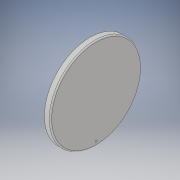
# Autodesk Inventor part: wheel hubcap
Saved by Autodesk Inventor 2019 (Build 230136000, 136)
## iProperties
Created: 2017-10-16
Part Number: wheel hubcap
Material: Generic
Document SubType Name: Modeling
Designer: M Koeppen
Density: 1 g/cm^3
Appearance: Default
Author: M Koeppen
Autodesk Inventor part; units mm, degrees
ref_plane "YZ Plane" through (0, 0, 0) normal (1, 0, 0) x (0, 1, 0)
ref_plane "XZ Plane" through (0, 0, 0) normal (0, 1, 0) x (-1, 0, 0)
ref_plane "XY Plane" through (0, 0, 0) normal (0, 0, 1) x (1, 0, 0)
sketch "Sketch5" plane through (0, 0, 0) normal (0, 0, 1) x (1, 0, 0)
  line L0 (0, 0) -> (0, 3.175)
  line L1 (0, 3.175) -> (5.715, 3.175)
  line L2 (6.35, 4.191) -> (6.35, 47.625)
  line L3 (6.35, 47.625) -> (12.7, 47.625)
  line L4 (12.7, 47.625) -> (12.7, 0)
  line L5 (12.7, 0) -> (0, 0)
  line L6 (5.715, 3.175) -> (5.715, 4.191)
  line L7 (5.715, 4.191) -> (6.35, 4.191)
  point P0 (9.525, 3.175)
  dimension "d9" = 3.175
  dimension "d10" = 47.625
  dimension "d14" = 6.35
  dimension "d18" = 0.635
  dimension "d19" = 4.191
  dimension "d21" = 5.715
  constraints: 16 end point, 5 perpendicular, 2 vertical, 1 point on line
  measures "d9" distance between parallel lines of L5 L1
  measures "d10" distance between parallel lines of L5 L3
  measures "d14" distance between parallel lines of L4 L2
  measures "d18" distance between parallel lines of L6 L2
  measures "d19" distance between parallel lines of L7 L5
  measures "d21" distance between parallel lines of L6 L0
revolve "Revolution1" add sketch "Sketch5" angle 360 about axis through (12.7, 0, 0) along (-1, 0, 0)
fillet "Fillet1" radius 1.27 1 edges at (12.7, -47.625, 0)
chamfer "Chamfer1" distance 0.635 angle 45 1 edges at (0, -3.175, 0)
sketch "Sketch6" plane through (12.7, 0, 0) normal (1, 0, 0) x (0, 0, -1)
  circle A0 centre (0, 0) radius 46.355 projected
  line L0 (-34.925, -19.05) -> (34.925, -19.05)
  line L1 (0, 0) -> (0, -19.05)
  point P0 (0, -43.18)
  dimension "d27" = 43.18
  dimension "d43" = 69.85
  dimension "d44" = 19.05
  constraints: 4 end point, 1 horizontal, 1 vertical
  measures "d27" distance of point (0, -43.18) L1.start
  measures "d43" distance of L0.start L0.end
  measures "d44" distance of L1.start L1.end
hole "Hole1" at (12.7, -43.18, 0) direction (-1, 0, 0) diameter 1.524 end through all
sketch "Sketch7" plane through (0, 0, 0) normal (-1, 0, 0) x (0, 0, 1)
  point P0 (0, 0)
hole "Hole2" at (0, 0, 0) direction (1, 0, 0) diameter 2.6416 depth 10.9728 tip angle 118 thread size "6-32 UNC" class "2B" standard "ANSI Unified Screw Threads"
body "Solid2"
